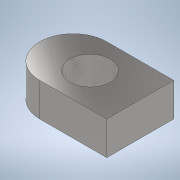
# Autodesk Inventor part: Pieza1
Saved by Autodesk Inventor 2021 (Build 250183000, 183)
## iProperties
Created: 2021-07-30
Part Number: Pieza1
Material: Acero inoxidable
Document SubType Name: Modeling
Designer: uriel
Density: 8 g/cm^3
Appearance: Semipulido
Author: uriel
Autodesk Inventor part; units mm, degrees
ref_plane "YZ Plane" through (0, 0, 0) normal (1, 0, 0) x (0, 1, 0)
ref_plane "XZ Plane" through (0, 0, 0) normal (0, 1, 0) x (-1, 0, 0)
ref_plane "XY Plane" through (0, 0, 0) normal (0, 0, 1) x (1, 0, 0)
sketch "Boceto1" plane through (0, 0, 0) normal (0, 1, 0) x (-1, 0, 0)
  line L0 (7.5, 5) -> (-7.5, 5)
  line L1 (-7.5, 5) -> (-7.5, -5)
  line L2 (-7.5, -5) -> (7.5, -5)
  line L3 (7.5, -5) -> (7.5, 5)
  line L4 (7.5, 5) -> (-7.5, -5) construction
  line L5 (-7.5, 5) -> (7.5, -5) construction
  circle A0 centre (0, 0) radius 3
  dimension "d0" = 15
  dimension "d1" = 10
  dimension "d2" = 6
  constraints: 12 end point, 2 midpoint, 2 parallel, 1 centre point, 1 coincident, 1 horizontal, 1 perpendicular
  measures "d0" distance of L2.end L1.end
  measures "d1" distance of L1.end L0.end
  measures "d2" diameter of A0
extrude "Extrusión1" add sketch "Boceto1" along normal mid plane 5
fillet "Empalme1" radius 5 2 edges at (-7.5, 0, 5) (-7.5, 0, -5)
